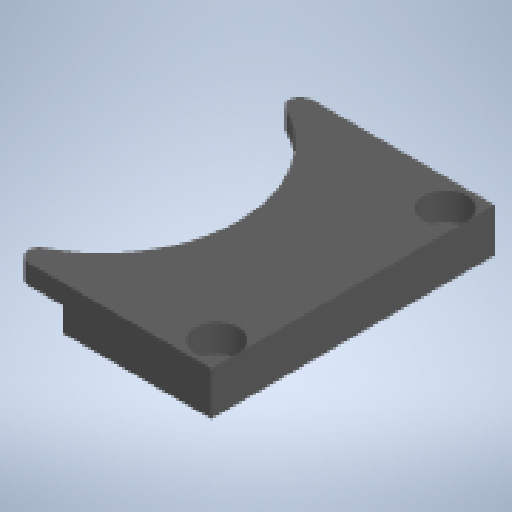
# Autodesk Inventor part: joit_cover
Saved by Autodesk Inventor 2024.1 (Build 281209000, 209)
## iProperties
Created: 2024-02-14
Part Number: joit_cover
Material: 一般
Document SubType Name: Modeling
Designer: hibik
Density: 1 g/cm^3
Appearance: 既定
Author: hibik
Autodesk Inventor part; units mm, degrees
ref_plane "YZ Plane" through (0, 0, 0) normal (1, 0, 0) x (0, 1, 0)
ref_plane "XZ Plane" through (0, 0, 0) normal (0, 1, 0) x (-1, 0, 0)
ref_plane "XY Plane" through (0, 0, 0) normal (0, 0, 1) x (1, 0, 0)
sketch "スケッチ1" plane through (0, 0, 0) normal (0, 1, 0) x (-1, 0, 0)
  line L0 (24, 0) -> (0, 0)
  line L1 (0, 0) -> (0, -26)
  line L2 (0, -26) -> (24, -26)
  line L3 (24, -26) -> (24, 0)
  circle A0 centre (24, -13) radius 13 construction
  circle A1 centre (24, -13) radius 12.5
  circle A2 centre (24, -13) radius 16
  point P0 (24, -25.5)
  point P1 (24, -0.5)
  point P2 (14.6726, 0)
  point P3 (14.6726, -26)
  dimension "d0" = 26
  dimension "d1" = 24
  dimension "d2" = 25
  dimension "d3" = 32
  constraints: 8 end point, 3 centre point, 3 coincident, 2 parallel, 1 horizontal, 1 midpoint, 1 perpendicular, 1 tangent
  measures "d0" distance of L2.end L0.start
  measures "d1" distance of L1.end L2.end
  measures "d2" diameter of A1
  measures "d3" diameter of A2
extrude "押し出し1" add sketch "スケッチ1" along normal blind 4 contours L3 A1 L2 A2 L0 | A2 L2 L1 L0 picked at (14.0879, -23.9339)
extrude "押し出し2" cut sketch "スケッチ1" along normal blind 2.2 contours L3 A1 L2 A2 L0 picked at (14.0879, -23.9339)
fillet "フィレット1" radius 1 4 edges at (-24, 3.1, -0.5) (-24, 3.1, 0) (-24, 3.1, -26) (-24, 3.1, -25.5)
sketch "スケッチ2" plane through (0, 4, 0) normal (0, 1, 0) x (1, 0, 0)
  circle A0 centre (-3, 2.5) radius 0.85 construction
  circle A1 centre (-3, 23.5) radius 0.85 construction
  circle A2 centre (-3, 2.5) radius 0.8
  circle A3 centre (-3, 23.5) radius 0.8
  point P0 (0, 0)
  dimension "d9" = 1.6
  dimension "d10" = 1.6
  constraints: 2 centre point, 2 coincident
  measures "d9" diameter of A2
  measures "d10" diameter of A3
extrude "押し出し3" cut sketch "スケッチ2" against normal through all
sketch "スケッチ4" plane through (0, 4, 0) normal (0, 1, 0) x (1, 0, 0)
  line L0 (0, 26) -> (-17.8153, 26) projected
  line L1 (0, 0) -> (-1, 0)
  line L2 (-1, 0) -> (-1, 26)
  line L3 (-1, 26) -> (0, 26)
  line L4 (0, 26) -> (0, 0)
  dimension "d20" = 1
  constraints: 8 end point, 2 parallel, 1 horizontal, 1 perpendicular, 1 point on line
  measures "d20" distance between parallel lines of L4 L2
extrude "押し出し5" cut sketch "スケッチ4" against normal through all
sketch "スケッチ3" plane through (0, 4, 0) normal (0, 1, 0) x (1, 0, 0)
  circle A0 centre (-3, 2.5) radius 0.8 projected
  circle A1 centre (-3, 23.5) radius 0.8 projected
  circle A2 centre (-3, 2.5) radius 2
  circle A3 centre (-3, 23.5) radius 2
  point P0 (0, 0)
  dimension "d13" = 4
  dimension "d14" = 4
  constraints: 2 centre point, 2 coincident
  measures "d13" diameter of A2
  measures "d14" diameter of A3
fillet "フィレット3" radius 2 3 edges at (-1, 4, -13) (-1, 2, 0) (-1, 2, -26)
extrude "押し出し6" cut sketch "スケッチ3" against normal blind 2
